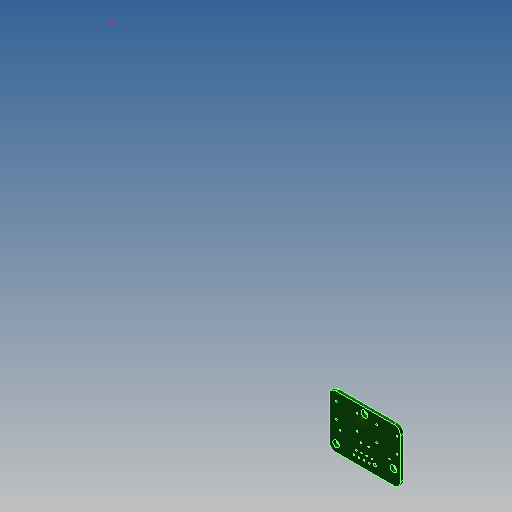
# Autodesk Inventor part: Manette_2019_PCB_Central.kicad_pcb_Contour
Saved by Autodesk Inventor 2019 (Build 230136000, 136)
## iProperties
Created: 2019-05-20
Part Number: Manette_2019_PCB_Central.kicad_pcb_Contour
Project: Nom Projet
Material: .
Description: Nom pièce
Document SubType Name: Modeling
Designer: Adel.KAHRIMANOVIC
Authority: brut Ø
Density: 0.001 g/cm^3
Appearance: Contour du circuit imprimé
Author: Adel.KAHRIMANOVIC
Material number: ---
Autodesk Inventor part; units mm, degrees
ref_plane "Plan YZ" through (0, 0, 0) normal (1, 0, 0) x (0, 1, 0)
ref_plane "Plan XZ" through (0, 0, 0) normal (0, 1, 0) x (-1, 0, 0)
ref_plane "Plan XY" through (0, 0, 0) normal (0, 0, 1) x (1, 0, 0)
sketch "Esquisse1" plane through (0, 0, 0) normal (0, 0, 1) x (1, 0, 0)
  point P0 (0, 0)
sketch "Esquisse6" plane through (0, 0, 0) normal (0, 0, 1) x (1, 0, 0)
  arc A0 (111.379, -99.822) -> (108.204, -102.997) centre (111.379, -102.997) ccw
  line L0 (108.204, -102.997) -> (108.204, -122.682)
  arc A1 (108.204, -122.682) -> (111.379, -125.857) centre (111.379, -122.682) ccw
  line L1 (111.379, -125.857) -> (139.954, -125.857)
  arc A2 (139.954, -125.857) -> (143.129, -122.682) centre (139.954, -122.682) ccw
  line L2 (143.129, -122.682) -> (143.129, -102.997)
  arc A3 (143.129, -102.997) -> (139.954, -99.822) centre (139.954, -102.997) ccw
  line L3 (139.954, -99.822) -> (111.379, -99.822)
  circle A4 centre (120.269, -122.428) radius 0.4
  circle A5 centre (121.539, -119.888) radius 0.4
  circle A6 centre (122.809, -122.428) radius 0.4
  circle A7 centre (124.079, -119.888) radius 0.4
  circle A8 centre (125.349, -122.428) radius 0.4
  circle A9 centre (126.619, -119.888) radius 0.4
  circle A10 centre (127.889, -122.428) radius 0.4
  circle A11 centre (129.159, -119.888) radius 0.4
  circle A12 centre (137.795, -115.57) radius 0.4
  circle A13 centre (127.635, -115.57) radius 0.4
  circle A14 centre (123.825, -115.57) radius 0.4
  circle A15 centre (113.665, -115.57) radius 0.4
  circle A16 centre (131.445, -111.76) radius 0.4
  circle A17 centre (141.605, -111.76) radius 0.4
  circle A18 centre (131.445, -104.14) radius 0.4
  circle A19 centre (141.605, -104.14) radius 0.4
  circle A20 centre (111.76, -111.76) radius 0.4
  circle A21 centre (121.92, -111.76) radius 0.4
  circle A22 centre (111.76, -104.14) radius 0.4
  circle A23 centre (121.92, -104.14) radius 0.4
  circle A24 centre (130.559, -121.688) radius 0.75
  circle A25 centre (139.7, -118.745) radius 1.6
  circle A26 centre (125.476, -102.616) radius 1.6
  circle A27 centre (111.633, -122.174) radius 1.6
  constraints: 28 centre point, 8 end point, 8 point on circle
extrude "Manette_2019_PCB_Central.kicad_pcb_Contour" add sketch "Esquisse6" along normal blind 1.6
